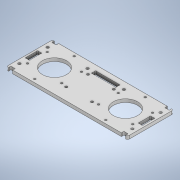
# Autodesk Inventor part: Trunk_waisit_frame_
Saved by Autodesk Inventor 2020.4 (Build 244396000, 396)
## iProperties
Created: 2021-12-30
Part Number: Trunk_waisit_frame_
Material: アルミニウム 2014-T4
Document SubType Name: Modeling
Designer: Masato Kubotera
Density: 2.8 g/cm^3
Appearance: 滑らか - 淡い灰色
Mass: 68.4365 g
Surface Area: 159.233 cm^2
Volume: 24.4416 cm^3
Description: A2017 T4
Author: Masato Kubotera
Autodesk Inventor part; units mm, degrees
ref_plane "YZ Plane" through (0, 0, 0) normal (1, 0, 0) x (0, 1, 0)
ref_plane "XZ Plane" through (0, 0, 0) normal (0, 1, 0) x (-1, 0, 0)
ref_plane "XY Plane" through (0, 0, 0) normal (0, 0, 1) x (1, 0, 0)
derived "Outer_support_stand.ipt"
sketch "スケッチ1" plane through (0, 0, 0) normal (0, 0, 1) x (1, 0, 0)
  circle A0 centre (0, 0) radius 18.5 construction
  circle A1 centre (0, 0) radius 20.5 construction
  circle A2 centre (0, 0) radius 20.51 construction
  line L0 (0, 0) -> (0, 24.5) construction
  circle A3 centre (0, 24.5) radius 1.55 construction
  circle A4 centre (0, 24.5) radius 3 construction
  arc A5 (0, 28.5) -> (-3.7147, 25.9835) centre (0, 24.5) ccw construction
  arc A6 (-5.1639, 24.7674) -> (-18.8673, 16.8557) centre (0, 0) ccw construction
  arc A7 (-5.1639, 24.7674) -> (-3.7147, 25.9835) centre (-5.5721, 26.7253) ccw construction
  arc A8 (3.7147, 25.9835) -> (5.1639, 24.7674) centre (5.5721, 26.7253) ccw construction
  arc A9 (3.7147, 25.9835) -> (0, 28.5) centre (0, 24.5) ccw construction
  circle A10 centre (0, 24.5) radius 3.05 construction
  arc A11 (-24.0311, 7.9117) -> (-24.0311, -7.9117) centre (0, 0) ccw construction
  arc A12 (-24.0311, 7.9117) -> (-24.3598, 9.7747) centre (-25.9308, 8.5371) ccw construction
  arc A13 (-24.6817, 14.25) -> (-24.3598, 9.7747) centre (-21.2176, 12.25) ccw construction
  arc A14 (-20.645, 16.2088) -> (-24.6817, 14.25) centre (-21.2176, 12.25) ccw construction
  arc A15 (-20.645, 16.2088) -> (-18.8673, 16.8557) centre (-20.3588, 18.1882) ccw construction
  circle A16 centre (-21.2176, 12.25) radius 3.05 construction
  circle A17 centre (-21.2176, 12.25) radius 1.55 construction
  arc A18 (-18.8673, -16.8557) -> (-5.1639, -24.7674) centre (0, 0) ccw construction
  arc A19 (-18.8673, -16.8557) -> (-20.645, -16.2088) centre (-20.3588, -18.1882) ccw construction
  arc A20 (-24.6817, -14.25) -> (-20.645, -16.2088) centre (-21.2176, -12.25) ccw construction
  arc A21 (-24.3598, -9.7747) -> (-24.6817, -14.25) centre (-21.2176, -12.25) ccw construction
  arc A22 (-24.3598, -9.7747) -> (-24.0311, -7.9117) centre (-25.9308, -8.5371) ccw construction
  circle A23 centre (-21.2176, -12.25) radius 3.05 construction
  circle A24 centre (-21.2176, -12.25) radius 1.55 construction
  arc A25 (5.1639, -24.7674) -> (18.8673, -16.8557) centre (0, 0) ccw construction
  arc A26 (5.1639, -24.7674) -> (3.7147, -25.9835) centre (5.5721, -26.7253) ccw construction
  arc A27 (0, -28.5) -> (3.7147, -25.9835) centre (0, -24.5) ccw construction
  arc A28 (-3.7147, -25.9835) -> (0, -28.5) centre (0, -24.5) ccw construction
  arc A29 (-3.7147, -25.9835) -> (-5.1639, -24.7674) centre (-5.5721, -26.7253) ccw construction
  circle A30 centre (0, -24.5) radius 3.05 construction
  circle A31 centre (0, -24.5) radius 1.55 construction
  arc A32 (24.0311, -7.9117) -> (24.0311, 7.9117) centre (0, 0) ccw construction
  arc A33 (24.0311, -7.9117) -> (24.3598, -9.7747) centre (25.9308, -8.5371) ccw construction
  arc A34 (24.6817, -14.25) -> (24.3598, -9.7747) centre (21.2176, -12.25) ccw construction
  arc A35 (20.645, -16.2088) -> (24.6817, -14.25) centre (21.2176, -12.25) ccw construction
  arc A36 (20.645, -16.2088) -> (18.8673, -16.8557) centre (20.3588, -18.1882) ccw construction
  circle A37 centre (21.2176, -12.25) radius 3.05 construction
  circle A38 centre (21.2176, -12.25) radius 1.55 construction
  arc A39 (18.8673, 16.8557) -> (5.1639, 24.7674) centre (0, 0) ccw construction
  arc A40 (18.8673, 16.8557) -> (20.645, 16.2088) centre (20.3588, 18.1882) ccw construction
  arc A41 (24.6817, 14.25) -> (20.645, 16.2088) centre (21.2176, 12.25) ccw construction
  arc A42 (24.3598, 9.7747) -> (24.6817, 14.25) centre (21.2176, 12.25) ccw construction
  arc A43 (24.3598, 9.7747) -> (24.0311, 7.9117) centre (25.9308, 8.5371) ccw construction
  circle A44 centre (21.2176, 12.25) radius 3.05 construction
  circle A45 centre (21.2176, 12.25) radius 1.55 construction
sketch "スケッチ2" plane through (0, 0, 0) normal (0, 0, 1) x (1, 0, 0)
  line L0 (-119, 28.5) -> (31, 28.5)
  line L1 (31, 28.5) -> (31, -28.5)
  line L2 (31, -28.5) -> (-119, -28.5)
  line L3 (-119, -28.5) -> (-119, 28.5)
  line L4 (-119, 28.5) -> (31, -28.5) construction
  line L5 (31, 28.5) -> (-119, -28.5) construction
  line L6 (-119, 0) -> (31, 0) construction
  line L7 (-44, 28.5) -> (-44, -28.5) construction
  line L8 (23.5, 7.5) -> (28.5, 7.5) construction
  line L9 (28.5, 7.5) -> (28.5, -7.5) construction
  line L10 (28.5, -7.5) -> (23.5, -7.5) construction
  line L11 (23.5, -7.5) -> (23.5, 7.5) construction
  line L12 (23.5, 7.5) -> (28.5, -7.5) construction
  line L13 (28.5, 7.5) -> (23.5, -7.5) construction
  circle A0 centre (26, -17.5) radius 1.6
  line L14 (23.45, 7.55) -> (28.55, 7.55)
  line L15 (28.55, 7.55) -> (28.55, -7.55)
  line L16 (28.55, -7.55) -> (23.45, -7.55)
  line L17 (23.45, -7.55) -> (23.45, 7.55)
  line L18 (23.45, 7.55) -> (28.55, -7.55) construction
  line L19 (28.55, 7.55) -> (23.45, -7.55) construction
  arc A1 (24.9349, 7.55) -> (23.45, 6.0651) centre (24.1925, 6.8075) ccw
  line L20 (26, 7.5) -> (26, -7.5) construction
  line L21 (23.5, 0) -> (28.5, 0) construction
  arc A2 (28.55, 6.0651) -> (27.0651, 7.55) centre (27.8075, 6.8075) ccw
  arc A3 (23.45, -6.0651) -> (24.9349, -7.55) centre (24.1925, -6.8075) ccw
  arc A4 (27.0651, -7.55) -> (28.55, -6.0651) centre (27.8075, -6.8075) ccw
  circle A5 centre (0, 24.5) radius 1.55 construction
  circle A6 centre (-21.2176, 12.25) radius 1.55 construction
  circle A7 centre (-21.2176, -12.25) radius 1.55 construction
  circle A8 centre (0, -24.5) radius 1.55 construction
  circle A9 centre (21.2176, -12.25) radius 1.55 construction
  circle A10 centre (21.2176, 12.25) radius 1.55 construction
  circle A11 centre (0, 24.5) radius 1.25
  circle A12 centre (-21.2176, 12.25) radius 1.25
  circle A13 centre (-21.2176, -12.25) radius 1.25
  circle A14 centre (0, -24.5) radius 1.25
  circle A15 centre (21.2176, -12.25) radius 1.25
  circle A16 centre (21.2176, 12.25) radius 1.25
  circle A17 centre (26, 17.5) radius 1.6
  circle A18 centre (-114, -17.5) radius 1.6
  line L22 (-111.45, 7.55) -> (-116.55, 7.55)
  line L23 (-116.55, 7.55) -> (-116.55, -7.55)
  line L24 (-116.55, -7.55) -> (-111.45, -7.55)
  line L25 (-111.45, -7.55) -> (-111.45, 7.55)
  arc A19 (-111.45, 6.0651) -> (-112.9349, 7.55) centre (-112.1925, 6.8075) ccw
  arc A20 (-115.0651, 7.55) -> (-116.55, 6.0651) centre (-115.8075, 6.8075) ccw
  arc A21 (-112.9349, -7.55) -> (-111.45, -6.0651) centre (-112.1925, -6.8075) ccw
  arc A22 (-116.55, -6.0651) -> (-115.0651, -7.55) centre (-115.8075, -6.8075) ccw
  circle A23 centre (-88, 24.5) radius 1.25
  circle A24 centre (-66.7824, 12.25) radius 1.25
  circle A25 centre (-66.7824, -12.25) radius 1.25
  circle A26 centre (-88, -24.5) radius 1.25
  circle A27 centre (-109.2176, -12.25) radius 1.25
  circle A28 centre (-109.2176, 12.25) radius 1.25
  circle A29 centre (-114, 17.5) radius 1.6
  circle A30 centre (0, 0) radius 10.5 construction
  line L26 (0, 0) -> (0, 24.5) construction
  line L27 (-31, -16) -> (-31, 16) construction
  line L28 (-31, 16) -> (12, 16) construction
  line L29 (12, 16) -> (12, -16) construction
  line L30 (12, -16) -> (-31, -16) construction
  line L31 (-31, -16) -> (12, 16) construction
  line L32 (-31, 16) -> (12, -16) construction
  line L33 (-31, 0) -> (12, 0) construction
  line L34 (-31, -14.4) -> (-39.5, -14.4) construction
  line L35 (-39.5, -14.4) -> (-39.5, 14.4) construction
  line L36 (-31, 14.4) -> (-39.5, 14.4) construction
  line L37 (-1, -13.5) -> (-1, 13.5) construction
  line L38 (-1, 13.5) -> (-28, 13.5) construction
  line L39 (-28, 13.5) -> (-28, -13.5) construction
  line L40 (-28, -13.5) -> (-1, -13.5) construction
  line L41 (-1, -13.5) -> (-28, 13.5) construction
  line L42 (-1, 13.5) -> (-28, -13.5) construction
  circle A31 centre (-28, -13.5) radius 1.5
  circle A32 centre (-28, 13.5) radius 1.5
  circle A33 centre (-60, -13.5) radius 1.5
  circle A34 centre (-60, 13.5) radius 1.5
  circle A35 centre (0, 0) radius 15
  circle A36 centre (-28, -13.5) radius 2.75 construction
  circle A37 centre (-88, 0) radius 15
  line L43 (-59, 22) -> (-29, 22) construction
  line L44 (-29, 22) -> (-29, 17) construction
  line L45 (-29, 17) -> (-59, 17) construction
  line L46 (-59, 17) -> (-59, 22) construction
  line L47 (-59, 22) -> (-29, 17) construction
  line L48 (-29, 22) -> (-59, 17) construction
  line L49 (-59.05, 22.05) -> (-28.95, 22.05)
  line L50 (-28.95, 22.05) -> (-28.95, 16.95)
  line L51 (-28.95, 16.95) -> (-59.05, 16.95)
  line L52 (-59.05, 16.95) -> (-59.05, 22.05)
  line L53 (-59.05, 22.05) -> (-28.95, 16.95) construction
  line L54 (-28.95, 22.05) -> (-59.05, 16.95) construction
  arc A38 (-30.4349, 16.95) -> (-28.95, 18.4349) centre (-29.6925, 17.6925) ccw
  line L55 (-59, 19.5) -> (-29, 19.5) construction
  arc A39 (-28.95, 20.5651) -> (-30.4349, 22.05) centre (-29.6925, 21.3075) ccw
  circle A40 centre (-21.5, 19.5) radius 1.6
  arc A41 (-59.05, 18.4349) -> (-57.5651, 16.95) centre (-58.3075, 17.6925) ccw
  arc A42 (-57.5651, 22.05) -> (-59.05, 20.5651) centre (-58.3075, 21.3075) ccw
  circle A43 centre (-66.5, 19.5) radius 1.6
  circle A44 centre (-21.5, 19.5) radius 2.75 construction
  line L56 (23.45, -28.5) -> (23.45, -26.9349)
  arc A45 (24.9349, -25.45) -> (23.45, -26.9349) centre (24.1925, -26.1925) ccw
  line L57 (24.9349, -25.45) -> (27.0651, -25.45)
  line L58 (28.55, -28.5) -> (28.55, -26.9349)
  arc A46 (28.55, -26.9349) -> (27.0651, -25.45) centre (27.8075, -26.1925) ccw
  line L59 (23.5, -25.5) -> (28.5, -25.5) construction
  line L60 (23.5, -25.5) -> (23.5, -28.5)
  line L61 (28.5, -25.5) -> (28.5, -28.5)
  line L62 (23.45, 28.5) -> (23.45, 26.9349)
  arc A47 (23.45, 26.9349) -> (24.9349, 25.45) centre (24.1925, 26.1925) ccw
  line L63 (24.9349, 25.45) -> (27.0651, 25.45)
  line L64 (28.55, 28.5) -> (28.55, 26.9349)
  arc A48 (27.0651, 25.45) -> (28.55, 26.9349) centre (27.8075, 26.1925) ccw
  line L65 (-111.45, -28.5) -> (-111.45, -26.9349)
  arc A49 (-111.45, -26.9349) -> (-112.9349, -25.45) centre (-112.1925, -26.1925) ccw
  line L66 (-112.9349, -25.45) -> (-115.0651, -25.45)
  line L67 (-116.55, -28.5) -> (-116.55, -26.9349)
  arc A50 (-115.0651, -25.45) -> (-116.55, -26.9349) centre (-115.8075, -26.1925) ccw
  line L68 (-111.45, 28.5) -> (-111.45, 26.9349)
  arc A51 (-112.9349, 25.45) -> (-111.45, 26.9349) centre (-112.1925, 26.1925) ccw
  line L69 (-112.9349, 25.45) -> (-115.0651, 25.45)
  line L70 (-116.55, 28.5) -> (-116.55, 26.9349)
  arc A52 (-116.55, 26.9349) -> (-115.0651, 25.45) centre (-115.8075, 26.1925) ccw
  circle A53 centre (26, -17.5) radius 3 construction
  point P0 (-44, 0)
  point P1 (0, 28.5)
  point P2 (0, -28.5)
  point P3 (26, 0)
  point P4 (26, 0)
  point P5 (27.0651, -7.55)
  point P6 (24.9349, -7.55)
  point P7 (23.45, -6.0651)
  point P8 (27.0651, 7.55)
  point P9 (28.55, 6.0651)
  point P10 (28.55, -6.0651)
  point P11 (-115.0651, 7.55)
  point P12 (-111.45, -6.0651)
  point P13 (-112.9349, -7.55)
  point P14 (-115.0651, -7.55)
  point P15 (-116.55, -6.0651)
  point P16 (-116.55, 6.0651)
  point P17 (-9.5, 0)
  point P18 (-14.5, 0)
  point P19 (-44, 19.5)
  point P20 (-59.05, 18.4349)
  point P21 (-59.05, 20.5651)
  point P22 (-57.5651, 22.05)
  point P23 (-30.4349, 22.05)
  point P24 (-28.95, 20.5651)
  point P25 (-57.5651, 16.95)
  point P26 (26, -25.45)
  point P27 (23.45, -25.45)
  point P28 (26, -24.294)
  dimension "d5" = 5
  dimension "d6" = 15
  dimension "d7" = 3.2
  dimension "d14" = 0.05
  dimension "d15" = 0.05
  dimension "d16" = 1.05
  dimension "d25" = 2.5
  dimension "d26" = 2.5
  dimension "d27" = 2.5
  dimension "d28" = 2.5
  dimension "d29" = 2.5
  dimension "d30" = 2.5
  dimension "d40" = 21
  dimension "d43" = 57
  dimension "d45" = 90
  dimension "d46" = 44
  dimension "d47" = 43
  dimension "d48" = 32
  dimension "d49" = 28.8
  dimension "d50" = 8.5
  dimension "d51" = 9.5
  dimension "d52" = 27
  dimension "d53" = 27
  dimension "d54" = 3
  dimension "d55" = 8.5
  dimension "d56" = 180
  dimension "d58" = 35
  dimension "d59" = 30
  dimension "d60" = 8.5
  dimension "d61" = 5.5
  dimension "d63" = 30
  dimension "d64" = 5
  dimension "d65" = 17
  dimension "d66" = 1.05
  dimension "d67" = 0.05
  dimension "d68" = 0.05
  dimension "d69" = 3.2
  dimension "d70" = 45
  dimension "d71" = 5.5
  dimension "d72" = 67.5
  dimension "d73" = 2.5
  dimension "d74" = 150
  dimension "d75" = 1.05
  dimension "d76" = 3
  dimension "d77" = 0.05
  dimension "d78" = 6
  constraints: 140 end point, 76 symmetric about line, 48 centre point, 43 point on circle, 28 midpoint, 23 point on line, 16 parallel, 14 perpendicular, 11 coincident, 1 collinear, 1 horizontal, 31 other
  measures "d5" distance of L9.end L10.end
  measures "d6" distance of L8.end L9.end
  measures "d7" diameter of A0
  measures "d14" distance between parallel lines of L17 L11
  measures "d15" distance between parallel lines of L14 L8
  measures "d16" radius of A1
  measures "d25" diameter of A11
  measures "d26" diameter of A12
  measures "d27" diameter of A13
  measures "d28" diameter of A14
  measures "d29" diameter of A15
  measures "d30" diameter of A16
  measures "d40" diameter of A30
  measures "d43" distance of L0.end L1.end
  measures "d45" angle of L0 L26
  measures "d46" distance of A30.centre point (-44, 0)
  measures "d47" distance of L27.end L28.end
  measures "d48" distance of L28.end L29.end
  measures "d49" distance of L34.end L35.end
  measures "d50" distance of L34.start L34.end
  measures "d51" distance of A30.centre point (-9.5, 0)
  measures "d52" distance of L39.end L38.end
  measures "d53" distance of L38.end L37.end
  measures "d54" diameter of A31
  measures "d55" distance from line of point (-9.5, 0) L37
  measures "d56" angle of L26 L27
  measures "d58" distance of A0.centre A17.centre
  measures "d59" diameter of A35
  measures "d60" distance edge to line of A35 L11
  measures "d61" diameter of A36
  measures "d63" distance of L44.end L45.end
  measures "d64" distance of L43.end L44.end
  measures "d65" vertical distance of point (-44, 0) L45.end
  measures "d66" radius of A38
  measures "d67" horizontal distance of L50.end L44.end
  measures "d68" horizontal distance of L50.end L44.end
  measures "d69" diameter of A40
  measures "d70" distance of A40.centre A43.centre
  measures "d71" diameter of A44
  measures "d72" distance of point (-44, 0) L21.start
  measures "d73" distance of L6.end L21.end
  measures "d74" distance of L0.start L0.end
  measures "d75" radius of A45
  measures "d76" distance of L59.end L61.end
  measures "d77" distance between parallel lines of L59 L57
  measures "d78" diameter of A53
extrude "押し出し1" add sketch "スケッチ2" along normal blind 4 contours L0 L70 A52 L69 A51 L68 L62 A47 L63 A48 L64 L1 L2 L58 A46 L57 A45 L56 L65 A49 L66 A50 L67 L3
fillet "フィレット1" radius 2.5 4 edges at (31, 28.5, 2) (31, -28.5, 2) (-119, -28.5, 2) (-119, 28.5, 2)
equation "\"d15\" = d14"
